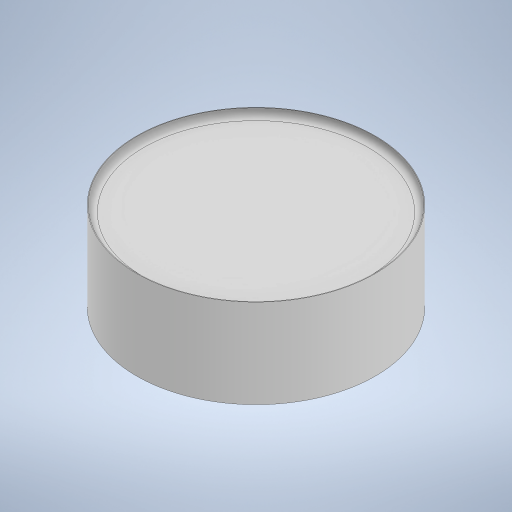
# Autodesk Inventor part: Module_bottom_Icicles25_v2
Saved by Autodesk Inventor 2023 (Build 270158000, 158)
## iProperties
Created: 2022-10-30
Part Number: Module_bottom_Icicles25_v2
Material: Generic
Document SubType Name: Modeling
Designer: incep
Density: 1 g/cm^3
Appearance: Default
Author: incep
## iProperties of the stored document Module_bottom_Icicles26_v2_3DPrint.ipt
Created: 2022-10-31
Part Number: Module_bottom_Icicles26_v2_3DPrint
Material: Generic
Document SubType Name: Modeling
Designer: incep
Density: 1 g/cm^3
Appearance: Default
Author: incep
Autodesk Inventor part; units mm, degrees
ref_plane "YZ Plane" through (0, 0, 0) normal (1, 0, 0) x (0, 1, 0)
ref_plane "XZ Plane" through (0, 0, 0) normal (0, 1, 0) x (-1, 0, 0)
ref_plane "XY Plane" through (0, 0, 0) normal (0, 0, 1) x (1, 0, 0)
sketch "Sketch3" plane through (0, 0, 0) normal (0, 1, 0) x (-1, 0, 0)
  circle A0 centre (0, 0) radius 18.4
  dimension "d32" = 36.8
  constraints: 1 centre point, 1 coincident
  measures "d32" diameter of A0
extrude "Extrusion4" add sketch "Sketch3" along normal blind 12.7
sketch "Sketch4" plane through (0, 12.7, 0) normal (0, 1, 0) x (1, 0, 0)
  circle A0 centre (0, 0) radius 18.4 projected
  circle A1 centre (0, 0) radius 17.75
  circle A2 centre (0, 0) radius 18.4 projected
  circle A3 centre (0, 0) radius 18.3
  dimension "d35" = 0.1
  constraints: 2 centre point, 2 coincident
  measures "d35" radial gap between concentric circles of A3 A0
sketch "Sketch4 outline for Extrusion5" plane through (0, 12.7, 0) normal (0, 1, 0) x (1, 0, 0)
  circle A0 centre (0, 0) radius 18.4
  circle A1 centre (0, 0) radius 18.3
extrude "Extrusion5" add sketch "Sketch4 outline for Extrusion5" along normal blind 1
fillet "Fillet1" radius 1 1 edges at (-18.3, 12.7, 0)
equation "\"d32\" = icicles25D"
equation "\"d33\" = chairThickness"
equation "\"moduleHeight\" = 96"
equation "\"moduleMountD\" = 6.8"
equation "\"moduleCornerR\" = 5"
equation "\"d4\" = moduleCornerR"
equation "\"d5\" = moduleMountD"
equation "\"d6\" = moduleMountD"
equation "\"d8\" = moduleMountD"
equation "\"d10\" = moduleMountD"
equation "\"moduleOpeningR\" = 25"
equation "\"d13\" = moduleOpeningR"
equation "\"thickness\" = 6"
equation "\"d15\" = thickness"
equation "\"d16\" = 0"
equation "\"iciclesMountD\" = 42.5"
equation "\"d17\" = iciclesMountD"
equation "\"clearanceM3\" = 3.6"
equation "\"d18\" = clearanceM6"
equation "\"d21\" = 360deg"
equation "\"d0\" = moduleHeight"
equation "\"iciclesBaseOuterD\" = 48"
equation "\"iciclesPlugD\" = 35.5"
equation "\"chairThickness\" = 12.7"
equation "\"isiclesBaseThickness\" = 3"
equation "\"clearanceM6\" = 3.6"
equation "\"d7\" = iciclesBaseOuterD"
equation "\"d9\" = iciclesMountD"
equation "\"d22\" = 360deg"
equation "\"d24\" = isiclesBaseThickness"
equation "\"d25\" = 0"
equation "\"d29\" = isiclesBaseThickness"
equation "\"compressedGasket\" = 0.5"
equation "\"d31\" = 0"
equation "\"iciclesPlugNeck\" = 16"
equation "\"headClearanceM3\" = 5.6"
equation "\"d42\" = 360deg"
equation "\"d45\" = 0"
equation "\"iciclesFilletR\" = 2"
equation "\"d46\" = iciclesFilletR"
equation "\"d47\" = iciclesFilletR"
equation "\"icicles25D\" = 36.8"
equation "\"icicles25T\" = 8.4"
equation "\"icicles25ND\" = 18"
equation "\"insertM3\" = 4"
equation "\"d11\" = insertM3"
equation "\"isiclesPlugT\" = icicles25T"
equation "\"d30\" = isiclesPlugT + chairThickness + compressedGasket"
equation "\"d39\" = headClearanceM3"
body "Solid2"
